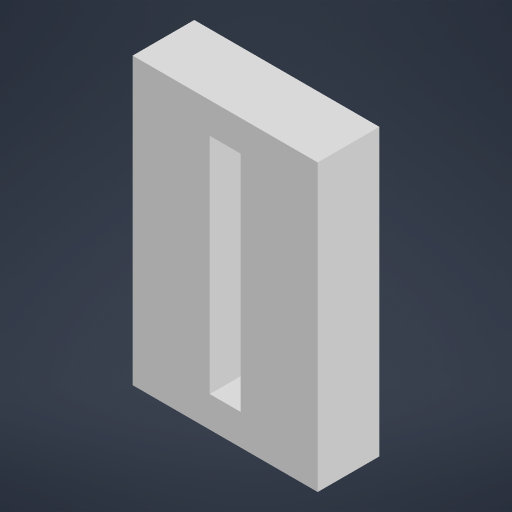
# Autodesk Inventor part: Rod
Saved by Autodesk Inventor 2024.1 (Build 281209000, 209)
## iProperties
Created: 2023-09-06
Part Number: Rod
Material: Generic
Document SubType Name: Modeling
Designer: User
Density: 1 g/cm^3
Appearance: Default
Author: User
Autodesk Inventor part; units mm, degrees
ref_plane "YZ Plane" through (0, 0, 0) normal (1, 0, 0) x (0, 1, 0)
ref_plane "XZ Plane" through (0, 0, 0) normal (0, 1, 0) x (-1, 0, 0)
ref_plane "XY Plane" through (0, 0, 0) normal (0, 0, 1) x (1, 0, 0)
sketch "Sketch12" plane through (0, 0, 0) normal (0, 0, 1) x (1, 0, 0)
  line L0 (0, 0) -> (-12, 0)
  line L1 (-12, 0) -> (-12, 18.5)
  line L2 (-12, 18.5) -> (0, 18.5)
  line L3 (0, 18.5) -> (0, 0)
  dimension "d50" = 12
  dimension "d51" = 18.5
  constraints: 8 end point, 2 parallel, 1 horizontal, 1 perpendicular
  measures "d50" distance of L1.end L2.end
  measures "d51" distance of L0.end L1.end
extrude "Extrusion8" add sketch "Sketch12" along normal blind 4
sketch "Sketch13" plane through (0, 0, 4) normal (0, 0, 1) x (1, 0, 0)
  line L0 (-12, 18.5) -> (-12, 0) projected
  line L1 (-12, 0) -> (-7, 0)
  line L2 (-7, 0) -> (-7, 2)
  line L3 (-7, 2) -> (-12, 2)
  line L4 (-12, 2) -> (-12, 0)
  line L5 (0, 18.5) -> (-12, 18.5) projected
  line L6 (0, 18.5) -> (-5, 18.5)
  line L7 (-5, 18.5) -> (-5, 16.5)
  line L8 (-5, 16.5) -> (0, 16.5)
  line L9 (0, 16.5) -> (0, 18.5)
  line L10 (-7, 2) -> (-5, 2)
  line L11 (-5, 2) -> (-5, 16.5)
  line L12 (-5, 16.5) -> (-7, 16.5)
  line L13 (-7, 16.5) -> (-7, 2)
  point P0 (0, 0)
  dimension "d54" = 5
  dimension "d55" = 2
  dimension "d56" = 5
  dimension "d57" = 2
  constraints: 24 end point, 6 parallel, 3 horizontal, 3 perpendicular
  measures "d54" distance of L3.end L2.end
  measures "d55" distance of L2.end L1.end
  measures "d56" distance of L8.end L7.end
  measures "d57" distance of L7.end L6.end
extrude "Extrusion9" cut sketch "Sketch13" against normal blind 4 contours L13 L12 L11 L10
body "Solid2"
